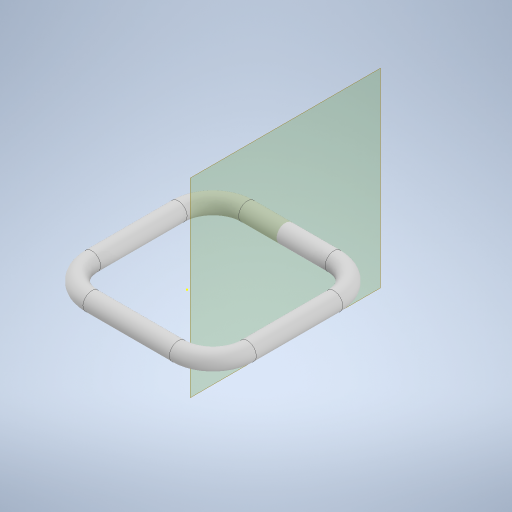
# Autodesk Inventor part: Деталь 8 лаба
Saved by Autodesk Inventor 2023.2 (Build 272271030, 271C)
## iProperties
Created: 2023-09-16
Part Number: Деталь 8 лаба
Material: Типовые
Document SubType Name: Modeling
Designer: User
Density: 1 g/cm^3
Appearance: По умолчанию
Author: User
Autodesk Inventor part; units mm, degrees
ref_plane "YZ Plane" through (0, 0, 0) normal (1, 0, 0) x (0, 1, 0)
ref_plane "XZ Plane" through (0, 0, 0) normal (0, 1, 0) x (-1, 0, 0)
ref_plane "XY Plane" through (0, 0, 0) normal (0, 0, 1) x (1, 0, 0)
sketch "Эскиз1" plane through (0, 0, 0) normal (0, 1, 0) x (-1, 0, 0)
  line L0 (4.3898, 6.6229) -> (-5.6102, 6.6229)
  line L1 (-9.6102, 2.6229) -> (-9.6102, -7.3771)
  line L2 (-5.6102, -11.3771) -> (4.3898, -11.3771)
  line L3 (8.3898, -7.3771) -> (8.3898, 2.6229)
  arc A0 (8.3898, 2.6229) -> (4.3898, 6.6229) centre (4.3898, 2.6229) ccw
  arc A1 (4.3898, -11.3771) -> (8.3898, -7.3771) centre (4.3898, -7.3771) ccw
  arc A2 (-9.6102, -7.3771) -> (-5.6102, -11.3771) centre (-5.6102, -7.3771) ccw
  arc A3 (-5.6102, 6.6229) -> (-9.6102, 2.6229) centre (-5.6102, 2.6229) ccw
  point P0 (0, 0)
  point P1 (-9.6102, -11.3771)
  point P2 (-9.6102, 6.6229)
  point P3 (8.3898, -11.3771)
  point P4 (0, -11.3771)
  dimension "d0" = 18
  dimension "d1" = 18
  dimension "d2" = 4
  constraints: 8 end point, 8 point on circle, 8 tangent, 7 point on line, 4 centre point, 3 equal radius, 2 parallel, 1 horizontal, 1 perpendicular
  measures "d0" distance of point (-9.61, -11.377) point (8.39, -11.377)
  measures "d1" distance of point (-9.61, 6.623) point (-9.61, -11.377)
  measures "d2" radius of A0
sketch "Эскиз2" plane through (0, 0, 0) normal (0, 1, 0) x (-1, 0, 0)
  point P0 (0, 0)
ref_plane "РабПлоскость1" through (0, 0, -11.3771) normal (-1, 0, 0) x (0, -1, 0)
sketch "Эскиз3" plane through (0, 0, -11.3771) normal (-1, 0, 0) x (0, -1, 0)
  circle A0 centre (0, 0) radius 1.0246
  point P0 (0, 11.3771)
  constraints: 1 centre point
sweep "Сдвиг1" add profiles "Эскиз3" path "Эскиз1"
